Autodesk Fusion 360 part; units mm, degrees
(part 2 of 2)
equation "PCB_Thickness = 1.78 mm"
equation "d71 = PCB_Thickness"
equation "d76 = MaterialThickness"
equation "d110 = MaterialThickness"
equation "d112 = -MaterialThickness"
equation "d114 = -MaterialThickness"
named bodies: "Bottom Shell", "PCB", "Lid"
